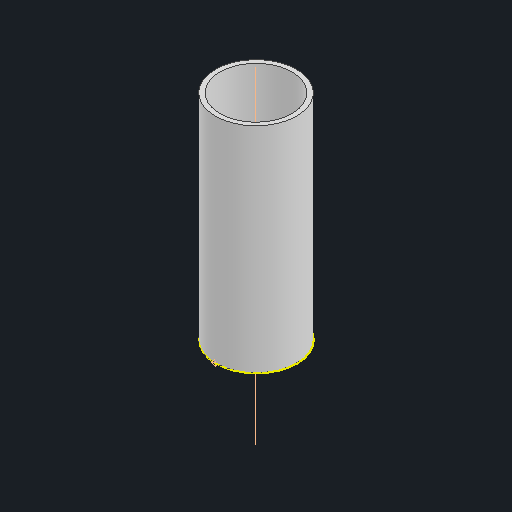
# Autodesk Inventor part: Coral
Saved by Autodesk Inventor 2024.3 (Build 283343010, 343A)
## iProperties
Created: 2025-03-08
Part Number: Coral
Material: Generic
Document SubType Name: Modeling
Designer: Owen L
Density: 1 g/cm^3
Appearance: Default
Author: Owen L
Autodesk Inventor part; units mm, degrees
ref_plane "YZ Plane" through (0, 0, 0) normal (1, 0, 0) x (0, 1, 0)
ref_plane "XZ Plane" through (0, 0, 0) normal (0, 1, 0) x (-1, 0, 0)
ref_plane "XY Plane" through (0, 0, 0) normal (0, 0, 1) x (1, 0, 0)
sketch "Sketch1" plane through (0, 0, 0) normal (0, 1, 0) x (-1, 0, 0)
  circle A0 centre (0, 0) radius 57.15
  circle A1 centre (0, 0) radius 50.8
  dimension "d0" = 114.3
  dimension "d1" = 101.6
  constraints: 2 centre point, 2 coincident
  measures "d0" diameter of A0
  measures "d1" diameter of A1
extrude "Extrusion1" add sketch "Sketch1" along normal blind 301.625
ref_plane "Work Plane1" through (0, 150.8125, 0) normal (0, -1, 0) x (1, 0, 0)
sketch "Sketch2" plane through (0, 0, 0) normal (0, -1, 0) x (1, 0, 0)
  circle A0 centre (0, 0) radius 57.15 projected
  line L0 (0, -57.15) -> (0, 57.15)
  constraints: 2 end point, 2 point on circle
body "Solid1"
